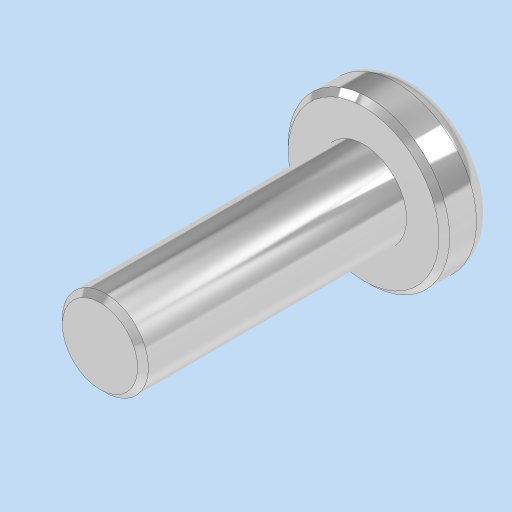
# Autodesk Inventor part: pan_head_screw_M1.6x5
Saved by Autodesk Inventor 2024 (Build 280153000, 153)
## iProperties
Created: 2025-05-11
Part Number: pan_head_screw_M1.6x5
Material: Nickel-Copper Alloy 400
Document SubType Name: Modeling
Designer: XxPan
Density: 8.83 g/cm^3
Appearance: Chrome - Polished
Author: XxPan
Autodesk Inventor part; units mm, degrees
ref_plane "YZ Plane" through (0, 0, 0) normal (1, 0, 0) x (0, 1, 0)
ref_plane "XZ Plane" through (0, 0, 0) normal (0, 1, 0) x (-1, 0, 0)
ref_plane "XY Plane" through (0, 0, 0) normal (0, 0, 1) x (1, 0, 0)
sketch "Sketch1" plane through (0, 0, 0) normal (0, 0, 1) x (1, 0, 0)
  circle A0 centre (0, 0) radius 1.5
  dimension "d0" = 3
  constraints: 1 centre point, 1 coincident
  measures "d0" diameter of A0
extrude "Extrusion1" add sketch "Sketch1" against normal blind 0.9
sketch "Sketch2" plane through (0, 0, 0) normal (0, 0, 1) x (1, 0, 0)
  circle A0 centre (0, 0) radius 1.5 projected
  circle A1 centre (0, 0) radius 0.8
  dimension "d3" = 1.6
  constraints: 1 centre point, 1 coincident
  measures "d3" diameter of A1
extrude "Extrusion2" add sketch "Sketch2" along normal blind 4.9 contours A1
fillet "Fillet1" radius 0.3 1 edges at (-1.5, 0, -0.9)
sketch "Sketch3" plane through (0, 0, -0.9) normal (0, 0, -1) x (-1, 0, 0)
  line L0 (-0.25, 0.25) -> (-0.25, 1)
  line L1 (-0.25, 1) -> (0.25, 1)
  line L2 (0.25, 1) -> (0.25, 0.25)
  line L3 (0.25, 0.25) -> (1, 0.25)
  line L4 (1, 0.25) -> (1, -0.25)
  line L5 (0.25, -0.25) -> (0.25, -1)
  line L6 (0.25, -1) -> (-0.25, -1)
  line L7 (-0.25, -1) -> (-0.25, -0.25)
  line L8 (-0.25, -0.25) -> (-1, -0.25)
  line L9 (-1, -0.25) -> (-1, 0.25)
  line L10 (-1, 0.25) -> (-0.25, 0.25)
  line L11 (0.25, -0.25) -> (1, -0.25)
  line L12 (2.1, 0) -> (-2.1, 0) construction
  line L13 (0, -2.1) -> (0, 2.1) construction
  point P0 (0, 0)
  dimension "d7" = 2
  dimension "d8" = 2
  dimension "d9" = 0.5
  constraints: 24 end point, 4 horizontal, 4 perpendicular, 3 collinear, 3 equal length, 3 vertical, 1 parallel, 1 point on line, 2 other
  measures "d7" distance between parallel lines of L6 L1
  measures "d8" distance between parallel lines of L4 L9
  measures "d9" distance of L0.end L1.end
extrude "Extrusion3" cut sketch "Sketch3" against normal blind 0.5
chamfer "Chamfer1" distance 0.1 angle 45 2 edges at (-1.5, 0, 0) (-0.8, 0, 4.9)
body "Solid1"
